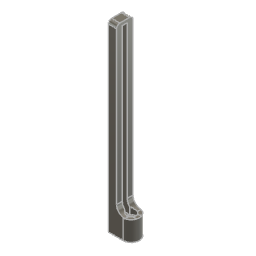
FinalCSProject4 v5 (Autodesk Fusion 360 design; units mm, degrees)
Autodesk Fusion 360 part; units mm, degrees
sketch "Sketch1" plane through (0, 0, 0) normal (0, 1, 0) x (1, 0, 0)
  circle A0 centre (0, 0) radius 1.6
  circle A1 centre (0, 0) radius 5
  dimension "d3" = 3.2
  dimension "d5" = 10
  constraint coincident A0.centre A1.centre
  measures "d3" diameter of A0
  measures "d5" diameter of A1
extrude "Extrude1" add sketch "Sketch1" along normal blind 4 contours A0 | A1
sketch "Sketch2" plane through (0, 4, 0) normal (0, 1, 0) x (-1, 0, 0)
  circle A0 centre (0, 0) radius 5
  circle A1 centre (0, 0) radius 1.6
  line L0 (-9, -5) -> (9, -5)
  line L1 (9, -5) -> (9, 5)
  line L2 (9, 5) -> (-9, 5)
  line L3 (-9, 5) -> (-9, -5)
  line L4 (-9, -5) -> (9, 5) construction
  line L5 (9, -5) -> (-9, 5) construction
  dimension "d8" = 3.2
  dimension "d11" = 18
  dimension "d12" = 10
  constraint horizontal L0
  constraint perpendicular L0 L1
  constraint parallel L0 L2
  constraint parallel L1 L3
  constraint coincident L4 A0.centre
  constraint coincident L5 A0.centre
  constraint coincident A0.centre A1.centre
  measures "d8" diameter of A1
  measures "d11" distance of L1.end L2.end
  measures "d12" distance of L0.end L1.end
extrude "Extrude2" add sketch "Sketch2" along normal blind 5 contours A0
extrude "Extrude14" add sketch "Sketch2" along normal blind 5 contours A0 L0 L1 L2
sketch "Sketch11" plane through (0, 9, 0) normal (0, 1, 0) x (-1, 0, 0)
  circle A0 centre (0, 0) radius 1.6
  arc A1 (0, 5) -> (0, -5) centre (0, 0) ccw
  line L0 (0, -5) -> (9, -5)
  line L1 (9, -5) -> (9, 5)
  line L2 (9, 5) -> (0, 5)
  line L3 (9, -5) -> (4, -5)
  line L4 (4, -5) -> (4, 5)
  line L5 (4, 5) -> (9, 5)
  line L6 (9, 5) -> (9, -5)
  dimension "d73" = 5
  constraint horizontal L3
  constraint vertical L4
  constraint horizontal L5
  constraint vertical L6
  constraint coincident L0.end L1.start
  measures "d73" distance of L0.end L3.end
extrude "Extrude15" add sketch "Sketch11" along normal blind 100 contours L0 L1 L2 L3 L4 L5 L6
sketch "Sketch12" plane through (-9, 0, 0) normal (-1, 0, 0) x (0, 0, 1)
  line L0 (-5, 4) -> (5, 4)
  line L1 (5, 4) -> (5, 109)
  line L2 (5, 109) -> (-5, 109)
  line L3 (-5, 109) -> (-5, 4)
  line L4 (-5, 109) -> (5, 4)
  line L5 (-5, 4) -> (5, 109)
  line L6 (1.5, 106.8727) -> (-1.5, 106.8727)
  line L7 (-1.5, 106.8727) -> (-1.5, 6.1273)
  line L8 (-1.5, 6.1273) -> (1.5, 6.1273)
  line L9 (1.5, 6.1273) -> (1.5, 106.8727)
  line L10 (1.5, 106.8727) -> (-1.5, 6.1273) construction
  line L11 (-1.5, 106.8727) -> (1.5, 6.1273) construction
  line L12 (1.6, 6) -> (-1.6, 6)
  line L13 (-1.6, 6) -> (-1.6, 107)
  line L14 (-1.6, 107) -> (1.6, 107)
  line L15 (1.6, 107) -> (1.6, 6)
  line L16 (1.6, 6) -> (-1.6, 107) construction
  line L17 (-1.6, 6) -> (1.6, 107) construction
  point P0 (0, 56.5)
  point P1 (0, 56.5)
  dimension "d76" = 3
  dimension "d95" = 3.2
  dimension "d96" = 101
  constraint coincident L2.end L3.start
  constraint coincident L0.end L1.start
  constraint coincident L0.start L3.end
  constraint coincident L1.end L2.start
  constraint horizontal L6
  constraint perpendicular L6 L7
  constraint parallel L6 L8
  constraint parallel L7 L9
  constraint coincident L10 P1
  constraint coincident L11 P1
  constraint midpoint L5 P1
  constraint horizontal L12
  constraint perpendicular L12 L13
  constraint parallel L12 L14
  constraint parallel L13 L15
  constraint coincident L16 P1
  constraint coincident L17 P1
  constraint coincident P1 P0
  measures "d76" distance of L7.end L8.end
  measures "d95" distance of L13.end L14.end
  measures "d96" distance of L12.end L13.end
extrude "Extrude16" cut sketch "Sketch12" against normal blind 100 contours L4 L5 L7 | L4 L5 L7 L8 L9 | L4 L5 L9 | L4 L5 L6 L7 L9
fillet "Fillet1" radius 2 1 edges at (-6.5, 109, 5)
sketch "Sketch13" plane through (0, 4, 0) normal (0, 1, 0) x (-1, 0, 0)
  circle A0 centre (0, 0) radius 2.75
  dimension "d81" = 5.5
  constraint coincident A0.centre origin
  measures "d81" diameter of A0
sketch "Sketch14" plane through (0, 9, 0) normal (0, 1, 0) x (-1, 0, 0)
  line L0 (0.5568, 1.5) -> (4, 1.5)
  line L1 (4, 1.5) -> (4, 5)
  line L2 (4, 5) -> (0, 5)
  arc A0 (0, 5) -> (-4.7697, 1.5) centre (0, 0) ccw
  line L3 (-4.7697, 1.5) -> (-0.5568, 1.5)
  arc A1 (0.5568, 1.5) -> (-0.5568, 1.5) centre (0, 0) ccw
  circle A2 centre (0, 0) radius 2.875
  dimension "d82" = 5.75
  constraint coincident A0.centre A1.centre
  measures "d82" diameter of A2
extrude "Extrude17" cut sketch "Sketch14" against normal blind 2.873 contours L0 L3 A1 A2 | L0 L3 A1 A2
fillet "Fillet2" radius 5 1 edges at (-4, 9, 3.25)
fillet "Fillet3" radius 5 1 edges at (-4, 9, -3.25)
extrude "Extrude18" add 1 faces at (4.2855, 6.1273, 0) along direction (0, 1, 0) blind 2.873
extrude "Extrude19" add sketch "Sketch2" against normal blind 4 contours A0 L0 L1 L2
fillet "Fillet4" radius 2 1 edges at (-6.5, 109, -5)
extrude "Extrude20" cut 1 faces at (-0.2445, 4, -0.1667) along direction (0, -1, 0) blind 100
extrude "Extrude21" add 1 faces at (-6.5333, 0, 0) along direction (0, -1, 0) blind 3
sketch "Sketch15" plane through (0, -3, 0) normal (0, -1, 0) x (1, 0, 0)
  circle A0 centre (0, 0) radius 1.6
  arc A1 (0, -5) -> (0, 5) centre (0, 0) ccw
  line L0 (0, 5) -> (-9, 5)
  line L1 (-9, 5) -> (-9, -5)
  line L2 (-9, -5) -> (0, -5)
  circle A2 centre (0, 0) radius 3.15
  dimension "d101" = 6.3
  constraint concentric A0 A2
  measures "d101" diameter of A2
extrude "Extrude22" cut sketch "Sketch15" against normal blind 3 contours A2
